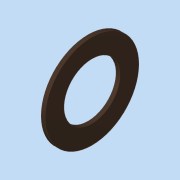
# Autodesk Inventor part: ThrustWasher
Saved by Autodesk Inventor 2017.3 (Build 213256000, 256)
## iProperties
Created: 2016-11-30
Part Number: ThrustWasher
Material: Bronze, Soft Tin
Document SubType Name: Modeling
Designer: techn
Density: 8.874 g/cm^3
Appearance: Bronze - Satin
Author: techn
Autodesk Inventor part; units mm, degrees
ref_plane "YZ Plane" through (0, 0, 0) normal (1, 0, 0) x (0, 1, 0)
ref_plane "XZ Plane" through (0, 0, 0) normal (0, 1, 0) x (-1, 0, 0)
ref_plane "XY Plane" through (0, 0, 0) normal (0, 0, 1) x (1, 0, 0)
sketch "Sketch1" plane through (0, 0, 0) normal (1, 0, 0) x (0, 1, 0)
  circle A0 centre (0, 0) radius 11.3792
  circle A1 centre (0, 0) radius 19.05
  dimension "d0" = 22.7584
  dimension "d1" = 38.1
  constraints: 2 centre point, 2 coincident
  measures "d0" diameter of A0
  measures "d1" diameter of A1
extrude "Extrusion1" add sketch "Sketch1" along normal blind 1.5875
body "Solid1"
